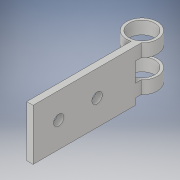
# Autodesk Inventor part: hinge half
Saved by Autodesk Inventor 2018 (Build 220112000, 112)
## iProperties
Created: 2019-01-18
Part Number: hinge half
Material: Generic
Document SubType Name: Modeling
Designer: s-2513225
Density: 1 g/cm^3
Appearance: Default
Author: s-2513225
Autodesk Inventor part; units mm, degrees
ref_plane "YZ Plane" through (0, 0, 0) normal (1, 0, 0) x (0, 1, 0)
ref_plane "XZ Plane" through (0, 0, 0) normal (0, 1, 0) x (-1, 0, 0)
ref_plane "XY Plane" through (0, 0, 0) normal (0, 0, 1) x (1, 0, 0)
sketch "Sketch1" plane through (0, 0, 0) normal (1, 0, 0) x (0, 1, 0)
  line L0 (0, 0) -> (25.4, 0)
  line L1 (25.4, 0) -> (25.4, -50.8)
  line L2 (25.4, -50.8) -> (0, -50.8)
  line L3 (0, -50.8) -> (0, 0)
  dimension "d0" = 25.4
  dimension "d1" = 50.8
  constraints: 8 end point, 2 parallel, 1 horizontal, 1 perpendicular
  measures "d0" distance of L1.end L2.end
  measures "d1" distance of L0.end L1.end
extrude "Extrusion1" add sketch "Sketch1" along normal blind 3.175
sketch "Sketch2" plane through (0, 25.4, 0) normal (0, 1, 0) x (1, 0, 0)
  line L0 (0, 50.8) -> (3.175, 50.8) projected
  arc A0 (3.175, 53.557) -> (0, 51.8122) centre (-1.9772, 59.1712) ccw
  line L1 (0, 50.8) -> (0, 0) projected
  line L2 (0, 50.8) -> (0, 51.8122)
  line L3 (3.175, 50.8) -> (3.175, 53.557)
  dimension "d4" = 15.24
  constraints: 4 end point, 2 point on circle, 1 centre point, 1 collinear, 1 parallel
  measures "d4" diameter of A0
extrude "Extrusion2" add sketch "Sketch2" against normal blind 6.35
ref_plane "Work Plane1" through (0, 9.525, 0) normal (0, -1, 0) x (1, 0, 0)
sketch "Sketch3" plane through (0, 9.525, 0) normal (0, -1, 0) x (1, 0, 0)
  arc A0 (0, -51.8122) -> (3.175, -53.557) centre (-1.9772, -59.1712) ccw projected
  line L0 (3.175, -53.557) -> (3.175, -50.8) projected
  line L1 (0, -50.8) -> (3.175, -50.8) projected
  line L2 (0, -50.8) -> (0, -51.8122) projected
  point P0 (0, 0)
extrude "Extrusion3" add sketch "Sketch3" along normal blind 6.35
sketch "Sketch4" plane through (0, 25.4, 0) normal (0, 1, 0) x (1, 0, 0)
  arc A0 (3.175, 53.557) -> (0, 51.8122) centre (-1.9772, 59.1712) ccw projected
  circle A1 centre (-1.9772, 59.1712) radius 6.35
  point P0 (0, 0)
  dimension "d10" = 12.7
  constraints: 1 centre point, 1 coincident
  measures "d10" diameter of A1
extrude "Extrusion4" cut sketch "Sketch4" against normal blind 127
sketch "Sketch5" plane through (3.175, 0, 0) normal (1, 0, 0) x (0, 0, -1)
  line L0 (0, 25.4) -> (0, 0) construction
  line L1 (0, 12.7) -> (12.7, 12.7) construction
  line L2 (12.7, 12.7) -> (31.75, 12.7) construction
  circle A0 centre (12.7, 12.7) radius 2.5797
  circle A1 centre (31.75, 12.7) radius 2.5797
  dimension "d13" = 12.7
  dimension "d14" = 19.05
  dimension "d15" = 5.1594
  dimension "d16" = 5.1594
  constraints: 4 end point, 2 centre point, 2 coincident, 1 horizontal, 1 midpoint, 1 point on line
  measures "d13" distance of L1.start L1.end
  measures "d14" distance of L1.end L2.end
  measures "d15" diameter of A0
  measures "d16" diameter of A1
extrude "Extrusion5" cut sketch "Sketch5" against normal blind 127
body "Solid1"
